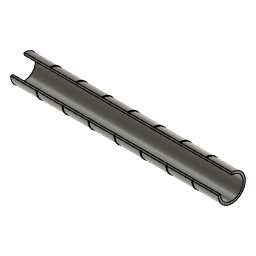
Front Array Greeblie (Autodesk Fusion 360 design; units mm, degrees)
Autodesk Fusion 360 part; units mm, degrees
sketch "Sketch1" plane through (0, 0, 0) normal (1, 0, 0) x (0, 1, 0)
  circle A0 centre (0, 0) radius 3.3
  circle A1 centre (0, 0) radius 2.75
  line L0 (0, 0) -> (-5, 0)
  line L1 (-5, 0) -> (-5, 5)
  line L2 (-5, 5) -> (0, 5)
  line L3 (0, 5) -> (0, 0)
  dimension "d1" = 6.6
  dimension "d39" = 5.5
  dimension "d42" = 5
  dimension "d43" = 5
  constraint coincident A0.centre A1.centre
  constraint concentric A0 A1
  constraint horizontal L0
  constraint vertical L1
  constraint horizontal L2
  constraint vertical L3
  measures "d1" diameter of A0
  measures "d39" diameter of A1
  measures "d42" distance of A0.centre L0.end
  measures "d43" distance of A0.centre L2.end
extrude "Extrude1" add sketch "Sketch1" along normal mid plane 50.6 contours A0 A1 L0 L3 | A0 A1 L0 L3 | A1 L0 L3 | A1 L0 L3
ref_plane "WorkPlane1" through (0, 0, 0) normal (1, 0, 0) x (0, 1, 0)
sketch "Sketch2" plane through (0, 0, 0) normal (1, 0, 0) x (0, 1, 0)
  circle A0 centre (0, 0) radius 3.3
  circle A1 centre (0, 0) radius 3.175
  dimension "d5" = 6.6
  dimension "d6" = 6.35
  constraint coincident A0.centre A1.centre
  constraint concentric A0 A1
  measures "d5" diameter of A0
  measures "d6" diameter of A1
extrude "Extrude2" cut sketch "Sketch2" along normal mid plane 0.25
ref_plane "WorkPlane2" through (12.65, 0, 0) normal (1, 0, 0) x (0, 1, 0)
sketch "Sketch3" plane through (12.65, 0, 0) normal (1, 0, 0) x (0, 1, 0)
  circle A0 centre (0, 0) radius 3.3
  circle A1 centre (0, 0) radius 3.175
  dimension "d10" = 6.6
  dimension "d11" = 6.35
  constraint coincident A0.centre A1.centre
  constraint concentric A0 A1
  measures "d10" diameter of A0
  measures "d11" diameter of A1
extrude "Extrude3" cut sketch "Sketch3" along normal mid plane 0.25
ref_plane "WorkPlane3" through (18.975, 0, 0) normal (1, 0, 0) x (0, 1, 0)
sketch "Sketch4" plane through (18.975, 0, 0) normal (1, 0, 0) x (0, 1, 0)
  circle A0 centre (0, 0) radius 3.3
  circle A1 centre (0, 0) radius 3.175
  dimension "d15" = 6.6
  dimension "d16" = 6.35
  constraint coincident A0.centre A1.centre
  constraint concentric A0 A1
  measures "d15" diameter of A0
  measures "d16" diameter of A1
extrude "Extrude4" cut sketch "Sketch4" along normal mid plane 0.25
ref_plane "WorkPlane4" through (6.325, 0, 0) normal (1, 0, 0) x (0, 1, 0)
sketch "Sketch5" plane through (6.325, 0, 0) normal (1, 0, 0) x (0, 1, 0)
  circle A0 centre (0, 0) radius 3.3
  circle A1 centre (0, 0) radius 3.175
  dimension "d20" = 6.6
  dimension "d21" = 6.35
  constraint coincident A0.centre A1.centre
  measures "d20" diameter of A0
  measures "d21" diameter of A1
extrude "Extrude5" cut sketch "Sketch5" along normal mid plane 0.25
ref_plane "WorkPlane5" through (-18.975, 0, 0) normal (-1, 0, 0) x (0, -1, 0)
sketch "Sketch6" plane through (-18.975, 0, 0) normal (-1, 0, 0) x (0, 1, 0)
  circle A0 centre (0, 0) radius 3.3
  circle A1 centre (0, 0) radius 3.175
  dimension "d25" = 6.6
  dimension "d26" = 6.35
  constraint coincident A0.centre A1.centre
  measures "d25" diameter of A0
  measures "d26" diameter of A1
extrude "Extrude6" cut sketch "Sketch6" along normal mid plane 0.25
ref_plane "WorkPlane6" through (-12.65, 0, 0) normal (-1, 0, 0) x (0, -1, 0)
sketch "Sketch7" plane through (-12.65, 0, 0) normal (-1, 0, 0) x (0, 1, 0)
  circle A0 centre (0, 0) radius 3.3
  circle A1 centre (0, 0) radius 3.175
  dimension "d30" = 6.6
  dimension "d31" = 6.35
  constraint coincident A0.centre A1.centre
  measures "d30" diameter of A0
  measures "d31" diameter of A1
extrude "Extrude7" cut sketch "Sketch7" along normal mid plane 0.25
ref_plane "WorkPlane7" through (-6.325, 0, 0) normal (-1, 0, 0) x (0, -1, 0)
sketch "Sketch8" plane through (-6.325, 0, 0) normal (-1, 0, 0) x (0, 1, 0)
  circle A0 centre (0, 0) radius 3.3
  circle A1 centre (0, 0) radius 3.175
  dimension "d35" = 6.6
  dimension "d36" = 6.35
  constraint coincident A0.centre A1.centre
  measures "d35" diameter of A0
  measures "d36" diameter of A1
extrude "Extrude8" cut sketch "Sketch8" along normal mid plane 0.25
extrude "Extrude9" cut sketch "Sketch1" along normal mid plane 60 contours A1 L0 L3 | A1 L0 L3
extrude "Extrude10" cut sketch "Sketch1" along normal mid plane 60 contours A0 A1 L0 L3 picked at (-3.1055, 0.1565)
